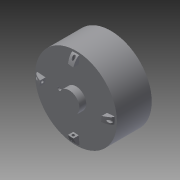
# Autodesk Inventor part: data_logger
Saved by Autodesk Inventor 2015 (Build 190159000, 159)
## iProperties
Created: 2019-09-28
Part Number: data_logger
Material: Generic
Document SubType Name: Modeling
Designer: gabri
Density: 1 g/cm^3
Appearance: Default
Author: gabri
Autodesk Inventor part; units mm, degrees
ref_plane "YZ Plane" through (0, 0, 0) normal (1, 0, 0) x (0, 1, 0)
ref_plane "XZ Plane" through (0, 0, 0) normal (0, 1, 0) x (-1, 0, 0)
ref_plane "XY Plane" through (0, 0, 0) normal (0, 0, 1) x (1, 0, 0)
sketch "Sketch2" plane through (0, 0, 0) normal (0, 0, 1) x (1, 0, 0)
  line L0 (0, -5) -> (-6, -5)
  line L1 (-6, -5) -> (-6, 0)
  line L2 (-30, -1.5) -> (-30, 0)
  line L3 (-7.5, -1.5) -> (-7.5, -6.5)
  line L4 (-7.5, -6.5) -> (0, -6.5)
  line L5 (-27, 0) -> (-27, 24)
  line L6 (-27, 24) -> (-30, 24)
  line L7 (-30, 24) -> (-30, 0)
  line L8 (-7.5, -1.5) -> (-30, -1.5)
  line L9 (-27, 0) -> (-6, 0)
  line L10 (0, -5) -> (0, -6.5)
  point P0 (0, 0)
  dimension "d16" = 1.5
  dimension "d18" = 1.5
  dimension "d21" = 3
  dimension "d22" = 24
  dimension "d51" = 5
  dimension "d52" = 1.5
  dimension "d53" = 1.5
  constraints: 22 end point, 2 parallel, 1 horizontal, 1 perpendicular, 1 vertical
  measures "d16" distance of L2.start L2.end
  measures "d18" distance between parallel lines of L3 L1
  measures "d21" distance of L5.end L6.end
  measures "d22" distance of L6.end L2.end
  measures "d51" distance between parallel lines of L9 L0
  measures "d52" distance between parallel lines of L8 L9
  measures "d53" distance of L0.start L4.end
revolve "Revolution1" add sketch "Sketch2" angle 360 about axis through (0, -5, 0) along (0, -1, 0)
sketch "Sketch4" plane through (0, 0, 0) normal (0, 1, 0) x (1, 0, 0)
  circle A0 centre (0, 0) radius 6 projected
  line L0 (-27, 1.5) -> (27, 1.5)
  line L1 (27, 1.5) -> (27, -1.5)
  line L2 (27, -1.5) -> (-27, -1.5)
  line L3 (-27, -1.5) -> (-27, 1.5)
  point P0 (0, 0)
  dimension "d28" = 1.5
  dimension "d29" = 3
  dimension "d30" = 27
  dimension "d31" = 27
  constraints: 8 end point, 2 parallel, 1 horizontal, 1 perpendicular
  measures "d28" distance from line of point (0, 0) L0
  measures "d29" distance of L0.end L1.end
  measures "d30" distance from line of point (0, 0) L3
  measures "d31" distance from line of point (0, 0) L1
extrude "Extrusion1" cut sketch "Sketch4" along normal blind 24 and the other way blind 0.5 contours A0 L2 L0 | A0 L0 L1 L2 | A0 L2 L3 L0
sketch "Sketch5" plane through (27, -0.5, -1.5) normal (-1, 0, 0) x (0, 0, 1)
  line L0 (3, 24.5) -> (0, 24.5)
  line L1 (0, 24.5) -> (0, 0.5)
  line L2 (0, 0.5) -> (3, 0.5)
  line L3 (3, 0.5) -> (3, 24.5)
  line L4 (31.5, 24.5) -> (-28.5, 24.5) projected
  point P0 (1.5, 0.5)
  point P1 (1.5, 0.5)
  dimension "d36" = 3
  dimension "d37" = 0
  constraints: 8 end point, 2 parallel, 1 coincident, 1 horizontal, 1 midpoint, 1 perpendicular
  measures "d36" distance of L1.end L2.end
  measures "d37" distance between parallel lines of L4 L0
extrude "Extrusion2" cut sketch "Sketch5" against normal blind 1
sketch "Sketch6" plane through (-27, -0.5, 1.5) normal (1, 0, 0) x (0, 0, -1)
  line L0 (0, 0.5) -> (3, 0.5)
  line L1 (3, 0.5) -> (3, 24.5)
  line L2 (3, 24.5) -> (0, 24.5)
  line L3 (0, 24.5) -> (0, 0.5)
  line L4 (31.5, 24.5) -> (-28.5, 24.5) projected
  point P0 (1.5, 0.5)
  point P1 (1.5, 0.5)
  point P2 (1.5, 24.5)
  dimension "d40" = 3
  constraints: 8 end point, 3 midpoint, 2 parallel, 1 coincident, 1 horizontal, 1 perpendicular
  measures "d40" distance between parallel lines of L1 L3
extrude "Extrusion3" cut sketch "Sketch6" against normal blind 1
sketch "Sketch7" plane through (0, -0.5, 0) normal (0, 1, 0) x (1, 0, 0)
  point P0 (0, 0)
  point P1 (-12, 0)
  dimension "d43" = 12
  measures "d43" distance of point (0, 0) point (-12, 0)
hole "Hole1" at (-12, -0.5, 0) direction (0, -1, 0) diameter 3 end through all
ref_plane "Work Plane1" through (-26.958301, 0, 0) normal (0, 0, 1) x (1, 0, 0)
sketch "Sketch10" plane through (-26.958301, 0, 0) normal (0, 0, 1) x (1, 0, 0)
  line L0 (56.958301, -1.5) -> (-3.041699, -1.5)
  line L1 (56.958301, -1.5) -> (-3.041699, -1.5)
  line L2 (26.958301, -1.5) -> (26.958301, -8)
  line L3 (-1.541699, -1.5) -> (0.458301, -1.5)
  line L4 (4.493832, -1.5) -> (4.493832, -5.5)
  ellipse E0 centre (26.958301, -1.5) end of major axis (-1.541699, -1.5) minor radius 6.5
  line L5 (0.458301, -1.5) -> (4.493832, -1.5)
  point P0 (26.958301, 0)
  dimension "d67" = 28.5
  dimension "d56" = 6.5
  dimension "d65" = 4
  constraints: 8 end point, 3 point on line, 2 vertical, 1 coincident, 1 collinear, 1 horizontal, 1 midpoint, 5 other
  measures "d56" distance of L2.start L2.end
  measures "d65" distance of L4.start L4.end
revolve "Revolution3" add sketch "Sketch10" angle 5 about axis through (0, -1.5, 0) along (0, -1, 0) and the other way 5 contours L4 E0 L0
sketch "Sketch12" plane through (-22.378985, -5.5, 1.957907) normal (0.0871557, 0, 0.9961947) x (0.9961947, 0, -0.0871557)
  line L0 (0, 4) -> (0.341286, 4)
  line L1 (0.341286, 4) -> (0.341286, 0)
  line L2 (0.341286, 0) -> (0, 0)
  line L3 (0, 0) -> (0, 4)
  point P0 (22.464469, 5.5)
  constraints: 8 end point, 2 parallel, 1 horizontal, 1 perpendicular
extrude "Extrusion5" cut sketch "Sketch12" against normal through all
pattern_circular "Circular Pattern1" count 4 over 360 about axis through (0, -4, 0) along (0, 1, 0) of "Revolution3", "Extrusion5"
sketch "Sketch14" plane through (0, -6.5, 0) normal (0, -1, 0) x (1, 0, 0)
  circle A0 centre (0, 0) radius 30
  line L0 (0, 0) -> (-29.127863, 4.630943)
  line L1 (-29.127863, 4.630943) -> (-29.127863, -4.440146)
  line L2 (-29.127863, -4.440146) -> (0, 0)
  line L3 (-28.268044, -3.439327) -> (-28.268044, 3.623625)
  line L4 (-29.127863, -4.440146) -> (-28.268044, -3.439327)
  line L5 (-28.268044, 3.623625) -> (-29.127863, 4.630943)
  point P0 (0, 0)
  dimension "d85" = 29.12786
  dimension "d86" = 29.12786
  constraints: 12 end point, 2 line through centre
  measures "d85" horizontal distance of L0.start L0.end
  measures "d86" horizontal distance of L1.end L0.start
extrude "Extrusion6" cut sketch "Sketch14" against normal up to surface (5 mm away) contours L5 L3 L4 L1
sketch "Sketch15" plane through (-28.268044, -2.105623, -2.473133) normal (-1, 0, 0) x (0, 0, 1)
  line L0 (0, 0) -> (0, 0.605623)
  line L1 (4.946267, 0.605623) -> (4.946267, 0)
  line L2 (4.946267, 0.605623) -> (0, 0.605623)
  line L3 (9.973133, -4.394377) -> (-5.026867, -4.394377)
  point P0 (2.473133, 2.105623)
  point P1 (2.473133, -1.394377)
  dimension "d89" = 2
  constraints: 1 horizontal alignment
  measures "d89" distance from line of L2 point (2.473, -1.394)
hole "Hole3" at (-28.268044, -3.5, 0) direction (1, 0, 0) diameter 2 depth 8 tip angle 118
pattern_circular "Circular Pattern2" count 4 over 360 about axis through (0, -4, 0) along (0, 1, 0) of "Hole3"
sketch "Sketch16" plane through (0, 24, 0) normal (0, 1, 0) x (1, 0, 0)
  circle A0 centre (0, 0) radius 30
  line L0 (-26.958301, -1.5) -> (-28, -1.5)
  line L1 (-28, -1.5) -> (-28, 1.5)
  line L2 (-28, 1.5) -> (-26.958301, 1.5)
  arc A1 (26.958301, 1.5) -> (-26.958301, 1.5) centre (0, 0) ccw
  line L3 (26.958301, 1.5) -> (28, 1.5)
  line L4 (28, 1.5) -> (28, -1.5)
  line L5 (28, -1.5) -> (26.958301, -1.5)
  arc A2 (-26.958301, -1.5) -> (26.958301, -1.5) centre (0, 0) ccw
  line L6 (0, 0) -> (6.359642, 40.025362)
  line L7 (0, 0) -> (-6.662481, 40.025362)
  line L8 (-6.662481, 40.025362) -> (6.359642, 40.025362)
  line L9 (-4.925918, 29.592826) -> (4.707654, 29.628331)
  circle A3 centre (0, 0) radius 30
  point P0 (0, 0)
  dimension "d103" = 40.02536
  dimension "d104" = 40.02536
  constraints: 8 end point, 2 point on line, 6 other
  measures "d103" vertical distance of L6.start L6.end
  measures "d104" vertical distance of L6.start L7.end
extrude "Extrusion7" cut sketch "Sketch16" against normal through all contours L9 A0 | A0 L7 L8 L6
pattern_circular "Circular Pattern3" count 6 over 360 about axis through (0, 12, 0) along (0, 1, 0) of "Extrusion7"
sketch "Sketch17" plane through (-4.925918, 24, -29.592826) normal (0, 1, 0) x (0.9999932, 0, -0.0036855)
  circle A0 centre (4.816819, -29.610779) radius 28.5
  line L0 (32.868915, -18.976877) -> (28.052097, -10.633902)
  arc A1 (28.052097, -10.633902) -> (9.633638, 0) centre (4.816819, -29.610779) ccw
  line L1 (9.633638, 0) -> (0, 0)
  arc A2 (0, 0) -> (-18.418459, -10.633902) centre (4.816819, -29.610779) ccw
  line L2 (-18.418459, -10.633902) -> (-23.235278, -18.976877)
  arc A3 (-23.235278, -18.976877) -> (-23.235278, -40.244682) centre (4.816819, -29.610779) ccw
  line L3 (-23.235278, -40.244682) -> (-18.418459, -48.587657)
  arc A4 (-18.418459, -48.587657) -> (0, -59.221559) centre (4.816819, -29.610779) ccw
  line L4 (0, -59.221559) -> (9.633638, -59.221559)
  arc A5 (9.633638, -59.221559) -> (28.052097, -48.587657) centre (4.816819, -29.610779) ccw
  line L5 (28.052097, -48.587657) -> (32.868915, -40.244682)
  arc A6 (32.868915, -40.244682) -> (32.868915, -18.976877) centre (4.816819, -29.610779) ccw
  line L6 (-22.146828, -31.011413) -> (-23.188519, -31.007574)
  line L7 (-23.188519, -31.007574) -> (-23.177463, -28.007595)
  line L8 (-23.177463, -28.007595) -> (-22.135771, -28.011434)
  arc A7 (31.780465, -28.210145) -> (-22.135771, -28.011434) centre (4.816819, -29.610779) ccw
  line L9 (31.780465, -28.210145) -> (32.822157, -28.213985)
  line L10 (32.822157, -28.213985) -> (32.8111, -31.213964)
  line L11 (32.8111, -31.213964) -> (31.769408, -31.210125)
  arc A8 (-22.146828, -31.011413) -> (31.769408, -31.210125) centre (4.816819, -29.610779) ccw
  circle A9 centre (4.816819, -29.610779) radius 28.5
  line L12 (0, 0) -> (9.633638, 0)
  line L13 (9.392797, -1.480539) -> (9.633638, 0)
  line L14 (0, 0) -> (0.240841, -1.480539)
  point P0 (4.816819, -29.610779)
  point P1 (4.711781, -58.110586)
  point P2 (7.405379, -1.228578)
  constraints: 6 end point, 3 point on circle, 1 centre point, 1 coincident, 1 collinear, 4 other
extrude "Extrusion8" add sketch "Sketch17" along normal blind 7 contours A0 L14 L1 L13
sketch "Sketch18" plane through (-4.925918, -1.5, -29.592826) normal (-0.0036855, 0, -0.9999932) x (-0.9999932, 0, 0.0036855)
  line L0 (-9.633638, 32.5) -> (0, 32.5)
  point P0 (-4.816819, 1.5)
  point P1 (-4.816819, 30)
  dimension "d112" = 2.5
  measures "d112" distance from line of L0 point (-4.817, 30)
hole "Hole4" at (-0.109132, 28.5, -29.610578) direction (0.0036855, 0, 0.9999932) diameter 2 depth 8 tip angle 118 countersink diameter 4.2 countersink angle 90
pattern_circular "Circular Pattern4" count 6 over 360 about axis through (0, 12, 0) along (0, 1, 0) of "Extrusion8", "Hole4"
equation "\"d18\" = d16"
equation "\"d29\" = 2 * d28"
equation "\"d86\" = d85"
equation "\"d104\" = d103"
body "Solid1"
